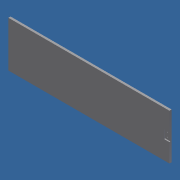
# Autodesk Inventor part: top panel for hinge
Saved by Autodesk Inventor 2012 (Build 160160000, 160)
## iProperties
Created: 2012-02-06
Part Number: top panel for hinge
Material: Default
Document SubType Name: Modeling
Designer: Allison Garza
Density: 1 g/cm^3
Author: Allison Garza
Autodesk Inventor part; units mm, degrees
ref_plane "YZ Plane" through (0, 0, 0) normal (1, 0, 0) x (0, 1, 0)
ref_plane "XZ Plane" through (0, 0, 0) normal (0, 1, 0) x (-1, 0, 0)
ref_plane "XY Plane" through (0, 0, 0) normal (0, 0, 1) x (1, 0, 0)
sketch "Sketch1" plane through (0, 0, 0) normal (0, 0, 1) x (1, 0, 0)
  line L0 (-35.8824, 13.1092) -> (434.0176, 13.1092)
  line L1 (434.0176, 13.1092) -> (434.0176, -120.2408)
  line L2 (434.0176, -120.2408) -> (-35.8824, -120.2408)
  line L3 (-35.8824, -120.2408) -> (-35.8824, 13.1092)
  point P0 (0, 0)
  dimension "d0" = 469.9
  dimension "d1" = 133.35
  constraints: 8 end point, 2 parallel, 1 horizontal, 1 perpendicular
  measures "d0" distance of L0.start L0.end
  measures "d1" distance of L2.end L0.start
extrude "Extrusion1" add sketch "Sketch1" along normal blind 6.35
sketch "Sketch2" plane through (0, 0, 6.35) normal (0, 0, 1) x (1, 0, 0)
  line L0 (434.0176, 13.1092) -> (434.0176, -120.2408) projected
  line L1 (434.0176, -40.8658) -> (418.1426, -40.8658)
  line L2 (418.1426, -40.8658) -> (418.1426, -66.2658)
  line L3 (418.1426, -66.2658) -> (434.0176, -66.2658)
  line L4 (434.0176, -66.2658) -> (434.0176, -40.8658)
  point P0 (0, 0)
  dimension "d4" = 15.875
  dimension "d5" = 25.4
  dimension "d6" = 53.975
  constraints: 8 end point, 2 parallel, 1 horizontal, 1 perpendicular, 1 point on line
  measures "d4" distance of L1.start L1.end
  measures "d5" distance of L1.end L2.end
  measures "d6" distance of L0.start L1.start
extrude "Extrusion2" cut sketch "Sketch2" against normal blind 3.175
sketch "Sketch3" plane through (0, 0, 3.175) normal (0, 0, 1) x (1, 0, 0)
  line L0 (418.1426, -40.8658) -> (418.1426, -66.2658) projected
  line L1 (434.0176, -40.8658) -> (418.1426, -40.8658) projected
  circle A0 centre (424.4926, -47.2158) radius 1.5875
  circle A1 centre (424.4926, -59.9158) radius 1.5875
  point P0 (0, 0)
  dimension "d9" = 12.7
  dimension "d10" = 6.35
  dimension "d11" = 6.35
  dimension "d12" = 3.175
  dimension "d13" = 3.175
  constraints: 2 centre point, 1 vertical alignment
  measures "d9" distance of A1.centre A0.centre
  measures "d10" distance from line of L1 A0.centre
  measures "d11" distance from line of A0.centre L0
  measures "d12" diameter of A0
  measures "d13" diameter of A1
extrude "Extrusion3" cut sketch "Sketch3" against normal blind 25.4
body "Solid1"
